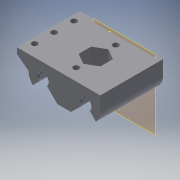
# Autodesk Inventor part: X Carriage
Saved by Autodesk Inventor 2016 (Build 200138000, 138)
## iProperties
Created: 2016-05-27
Part Number: X Carriage
Material: Generic
Document SubType Name: Modeling
Designer: Scott
Density: 1 g/cm^3
Appearance: Default
Author: Scott
Autodesk Inventor part; units mm, degrees
ref_plane "YZ Plane" through (0, 0, 0) normal (1, 0, 0) x (0, 1, 0)
ref_plane "XZ Plane" through (0, 0, 0) normal (0, 1, 0) x (-1, 0, 0)
ref_plane "XY Plane" through (0, 0, 0) normal (0, 0, 1) x (1, 0, 0)
ref_plane "Work Plane1" through (0, 0, 0) normal (0, 0, 1) x (1, 0, 0)
sketch "Sketch1" plane through (0, 0, 0) normal (0, 0, 1) x (1, 0, 0)
  circle A0 centre (31.455, -10.16) radius 4 projected
  circle A1 centre (-6.055, -10.16) radius 4 projected
  circle A2 centre (-6.055, -10.16) radius 8
  circle A3 centre (31.455, -10.16) radius 8
  circle A4 centre (-6.055, -10.16) radius 12.7
  circle A5 centre (31.455, -10.16) radius 12.7
  line L0 (-6.055, 2.54) -> (31.455, 2.54)
  line L1 (-6.055, -22.86) -> (31.455, -22.86)
  point P0 (0, 0)
  dimension "d0" = 16
  dimension "d1" = 16
  dimension "d2" = 25.4
  dimension "d3" = 25.4
  constraints: 4 centre point, 4 coincident, 4 end point, 4 point on circle, 2 tangent
  measures "d0" diameter of A2
  measures "d1" diameter of A3
  measures "d2" diameter of A4
  measures "d3" diameter of A5
extrude "Extrusion1" add sketch "Sketch1" along normal blind 24 contours A4 | A4 L0 A5 L1 | A5
sketch "Sketch2" plane through (-6.055, 2.54, 0) normal (0, 1, 0) x (1, 0, 0)
  point P0 (6.055, 0)
sketch "Sketch3" plane through (0, 0, 24) normal (0, 0, 1) x (1, 0, 0)
  circle A0 centre (31.455, -10.16) radius 8 projected
  circle A1 centre (-6.055, -10.16) radius 8 projected
  line L0 (-6.055, -22.86) -> (31.455, -22.86) projected
  arc A2 (31.455, -22.86) -> (31.455, 2.54) centre (31.455, -10.16) ccw projected
  line L1 (31.455, 2.54) -> (-6.055, 2.54) projected
  arc A3 (-6.055, 2.54) -> (-6.055, -22.86) centre (-6.055, -10.16) ccw projected
  circle A4 centre (-6.055, -10.16) radius 5
  circle A5 centre (31.455, -10.16) radius 5
  point P0 (0, 0)
  dimension "d6" = 10
  dimension "d7" = 10
  constraints: 2 centre point, 2 coincident
  measures "d6" diameter of A4
  measures "d7" diameter of A5
extrude "Extrusion2" add sketch "Sketch3" along normal blind 2 contours A0 | A1 | A3 L1 A2 L0
sketch "Sketch4" plane through (0, 0, 26) normal (0, 0, 1) x (1, 0, 0)
  circle A0 centre (-6.055, -10.16) radius 5 projected
  circle A1 centre (31.455, -10.16) radius 5 projected
  line L0 (-6.055, -22.86) -> (31.455, -22.86) projected
  arc A2 (31.455, -22.86) -> (31.455, 2.54) centre (31.455, -10.16) ccw projected
  line L1 (31.455, 2.54) -> (-6.055, 2.54) projected
  arc A3 (-6.055, 2.54) -> (-6.055, -22.86) centre (-6.055, -10.16) ccw projected
  circle A4 centre (-6.055, -10.16) radius 8 projected
  circle A5 centre (31.455, -10.16) radius 8 projected
  point P0 (0, 0)
extrude "Extrusion3" add sketch "Sketch4" along normal blind 24 contours A3 L1 A2 L0
sketch "Sketch5" plane through (-6.055, 2.54, 0) normal (0, 1, 0) x (1, 0, 0)
  line L0 (37.51, 0) -> (0, 0) projected
  line L1 (0, 0) -> (0, -50) projected
  line L2 (37.51, -50) -> (0, -50) projected
  line L3 (37.51, 0) -> (37.51, -50) projected
  circle A0 centre (18.755, -25) radius 6.5
  point P0 (6.055, 0)
  dimension "d12" = 13
  constraints: 1 centre point
  measures "d12" diameter of A0
extrude "Extrusion4" cut sketch "Sketch5" against normal blind 36.700003 contours A0
sketch "Sketch6" plane through (0, 0, 50) normal (0, 0, 1) x (1, 0, 0)
  circle A0 centre (31.455, -10.16) radius 8
  circle A1 centre (-6.055, -10.16) radius 8
  line L0 (-6.055, -22.86) -> (31.455, -22.86)
  arc A2 (31.455, -22.86) -> (31.455, 2.54) centre (31.455, -10.16) ccw
  line L1 (31.455, 2.54) -> (-6.055, 2.54)
  arc A3 (-6.055, 2.54) -> (-6.055, -22.86) centre (-6.055, -10.16) ccw
  circle A4 centre (-6.055, -10.16) radius 8
  line L2 (-11.774138, -15.753877) -> (-14.91362, -19.260266)
  arc A5 (-6.055, 2.54) -> (-6.055, -22.86) centre (-6.055, -10.16) ccw
  line L3 (-11.774138, -15.753877) -> (-7.067641, -15.753877) construction
  line L4 (-0.461123, -15.879138) -> (6.51974, -22.86)
  line L5 (-6.055, -22.86) -> (31.455, -22.86)
  line L6 (-0.461123, -15.879138) -> (9.411307, -15.879138) construction
  circle A6 centre (31.455, -10.16) radius 8
  line L7 (25.735862, -15.753877) -> (18.470616, -22.86)
  line L8 (37.048877, -15.879138) -> (40.33528, -19.239131)
  arc A7 (31.455, -22.86) -> (31.455, 2.54) centre (31.455, -10.16) ccw
  line L9 (25.735862, -15.753877) -> (31.455, -10.16)
  line L10 (31.455, -10.16) -> (37.048877, -15.879138)
  line L11 (-0.461123, -15.879138) -> (-6.055, -10.16)
  line L12 (-6.055, -10.16) -> (-11.774138, -15.753877)
  point P0 (0, 0)
  dimension "d16" = 45
  constraints: 20 end point, 11 point on circle, 4 perpendicular, 2 equal length, 2 horizontal, 2 point on line, 1 parallel
  measures "d16" angle of L4 L6
extrude "Extrusion5" cut sketch "Sketch6" against normal blind 96.8375 contours L9 L10 A0 | A0 L8 A2 L0 L7 | L0 A3 L2 A1 L4 | A1 L12 L11 picked at (31.396323, -15.459474) picked at (-8.407222, -14.909202)
sketch "Sketch7" plane through (0, 0, 0) normal (0, 0, -1) x (-1, 0, 0)
  line L0 (11.774138, -15.753877) -> (14.91362, -19.260266)
  arc A0 (14.91362, -19.260266) -> (6.055, 2.54) centre (6.055, -10.16) ccw
  line L1 (-31.455, 2.54) -> (6.055, 2.54)
  arc A1 (-31.455, 2.54) -> (-40.33528, -19.239131) centre (-31.455, -10.16) ccw
  line L2 (-40.33528, -19.239131) -> (-37.048877, -15.879138)
  arc A2 (-25.735862, -15.753877) -> (-37.048877, -15.879138) centre (-31.455, -10.16) ccw
  line L3 (-25.735862, -15.753877) -> (-18.470616, -22.86)
  line L4 (-6.51974, -22.86) -> (-18.470616, -22.86)
  line L5 (-6.51974, -22.86) -> (0.461123, -15.879138)
  arc A3 (11.774138, -15.753877) -> (0.461123, -15.879138) centre (6.055, -10.16) ccw
  arc A4 (-25.735862, -15.753877) -> (-37.048877, -15.879138) centre (-31.455, -10.16) ccw
  arc A5 (-27.880539, -13.656173) -> (-34.951173, -13.734461) centre (-31.455, -10.16) ccw
  line L6 (-37.048877, -15.879138) -> (-34.951173, -13.734461)
  arc A6 (-27.880539, -13.656173) -> (-34.951173, -13.734461) centre (-31.455, -10.16) ccw
  line L7 (-27.880539, -13.656173) -> (-25.735862, -15.753877)
  arc A7 (-25.735862, -15.753877) -> (-37.048877, -15.879138) centre (-31.455, -10.16) ccw
  line L8 (9.629461, -13.656173) -> (11.774138, -15.753877)
  arc A8 (11.774138, -15.753877) -> (0.461123, -15.879138) centre (6.055, -10.16) ccw
  line L9 (0.461123, -15.879138) -> (2.558827, -13.734461)
  arc A9 (9.629461, -13.656173) -> (2.558827, -13.734461) centre (6.055, -10.16) ccw
  point P0 (0, 0)
extrude "Extrusion6" add sketch "Sketch7" along normal blind 2.54
sketch "Sketch8" plane through (0, 0, 50) normal (0, 0, 1) x (1, 0, 0)
  line L0 (-14.91362, -19.260266) -> (-11.774138, -15.753877)
  arc A0 (-0.461123, -15.879138) -> (-11.774138, -15.753877) centre (-6.055, -10.16) ccw
  line L1 (-0.461123, -15.879138) -> (6.51974, -22.86)
  line L2 (6.51974, -22.86) -> (18.470616, -22.86)
  line L3 (18.470616, -22.86) -> (25.735862, -15.753877)
  arc A1 (37.048877, -15.879138) -> (25.735862, -15.753877) centre (31.455, -10.16) ccw
  line L4 (37.048877, -15.879138) -> (40.33528, -19.239131)
  arc A2 (40.33528, -19.239131) -> (31.455, 2.54) centre (31.455, -10.16) ccw
  line L5 (31.455, 2.54) -> (-6.055, 2.54)
  arc A3 (-6.055, 2.54) -> (-14.91362, -19.260266) centre (-6.055, -10.16) ccw
  line L6 (-11.774138, -15.753877) -> (-9.629461, -13.656173)
  arc A4 (-2.558827, -13.734461) -> (-9.629461, -13.656173) centre (-6.055, -10.16) ccw
  line L7 (-2.558827, -13.734461) -> (-0.461123, -15.879138)
  arc A5 (-0.461123, -15.879138) -> (-11.774138, -15.753877) centre (-6.055, -10.16) ccw
  line L8 (34.951173, -13.734461) -> (37.048877, -15.879138)
  arc A6 (37.048877, -15.879138) -> (25.735862, -15.753877) centre (31.455, -10.16) ccw
  line L9 (25.735862, -15.753877) -> (27.880539, -13.656173)
  arc A7 (34.951173, -13.734461) -> (27.880539, -13.656173) centre (31.455, -10.16) ccw
  point P0 (0, 0)
extrude "Extrusion7" add sketch "Sketch8" along normal blind 2.54
sketch "Sketch9" plane through (-6.055, 2.54, -2.54) normal (0, 1, 0) x (1, 0, 0)
  line L0 (50.21, 0) -> (50.21, -55.08) projected
  line L1 (37.51, 0) -> (37.51, -55.08) projected
  line L2 (50.21, 0) -> (37.51, 0) projected
  line L3 (37.51, -55.08) -> (50.21, -55.08) projected
  point P0 (6.055, -2.54)
  point P1 (46.39028, 0)
  point P2 (46.39028, -55.08)
extrude "Extrusion8" add sketch "Sketch9" against normal up to next
sketch "Sketch10" plane through (-6.055, 2.54, 52.54) normal (0, 1, 0) x (1, 0, 0)
  line L0 (5, 0) -> (-5, 0)
  line L1 (-8, 52.54) -> (8, 52.54)
  line L2 (-5.719138, 52.54) -> (-5.719138, 2.54)
  line L3 (-5.719138, 52.54) -> (44.280862, 52.54) construction
  circle A0 centre (18.755, 27.54) radius 6.5
  line L4 (0, 55.08) -> (0, 0)
  line L5 (50.21, 0) -> (0, 0)
  line L6 (50.21, 55.08) -> (50.21, 0)
  line L7 (0, 55.08) -> (50.21, 55.08)
  line L8 (-8.85862, 55.08) -> (-8.85862, 0)
  line L9 (0, 0) -> (-8.85862, 0)
  line L10 (0, 55.08) -> (0, 0)
  line L11 (-8.85862, 55.08) -> (0, 55.08)
  point P0 (6.055, 52.54)
  point P1 (-3.574461, 0)
  point P2 (3.496173, 0)
  point P3 (5.593877, 52.54)
  dimension "d25" = 90
  constraints: 4 end point, 1 horizontal, 1 perpendicular
  measures "d25" angle of L2 L3
extrude "Extrusion9" add sketch "Sketch10" against normal up to next contours L0 L9 L8 L11 L4
sketch "Sketch11" plane through (44.155, 2.54, 52.54) normal (0, 1, 0) x (1, 0, 0)
  line L0 (0, 55.08) -> (0, 0)
  line L1 (-4.7, 52.54) -> (-4.7, 28.54)
  line L2 (0, 55.08) -> (0, 0)
  line L3 (0, 0) -> (-59.06862, 0)
  line L4 (0, 55.08) -> (-3.81, 55.08)
  line L5 (-3.81, 55.08) -> (-3.81, 0)
  line L6 (-3.81, 0) -> (0, 0)
  line L7 (0, 0) -> (0, 55.08)
  point P0 (-44.155, 52.54)
  dimension "d28" = 3.81
  constraints: 8 end point, 2 parallel, 1 horizontal, 1 perpendicular, 1 point on line
  measures "d28" distance of L6.end L5.end
extrude "Extrusion10" add sketch "Sketch11" along normal blind 12.7
sketch "Sketch12" plane through (-14.91362, 2.54, 52.54) normal (0, 1, 0) x (1, 0, 0)
  line L0 (55.25862, 0) -> (55.25862, 55.08)
  line L1 (55.25862, 55.08) -> (0, 55.08)
  line L2 (0, 55.08) -> (0, 0)
  line L3 (55.25862, 0) -> (0, 0)
  circle A0 centre (27.61362, 27.54) radius 6.5
  circle A1 centre (27.61362, 27.54) radius 6.5
  line L4 (27.475496, 34.038532) -> (27.475496, 55.08)
  line L5 (33.384236, 55.08) -> (21.43336, 55.08)
  line L6 (27.475496, 34.038532) -> (48.516964, 34.038532) construction
  line L7 (27.478162, 21.041412) -> (27.478162, 0)
  line L8 (55.25862, 0) -> (0, 0)
  line L9 (27.478162, 21.041412) -> (48.519574, 21.041412) construction
  circle A2 centre (27.62931, 44.942828) radius 2.54
  circle A3 centre (27.478162, 10.520706) radius 2.54
  point P0 (14.91362, 52.54)
  dimension "d31" = 90
  dimension "d32" = 90
  dimension "d33" = 5.08
  dimension "d34" = 5.08
  constraints: 8 end point, 4 point on circle, 2 centre point, 2 horizontal, 2 perpendicular, 2 point on line, 1 midpoint
  measures "d31" angle of L6 L4
  measures "d32" angle of L7 L9
  measures "d33" diameter of A2
  measures "d34" diameter of A3
extrude "Extrusion11" cut sketch "Sketch12" against normal blind 76.2 contours A3 L7 | L7 A3 | A2 L4 | L4 A2
sketch "Sketch13" plane through (-14.91362, 2.54, 52.54) normal (0, 1, 0) x (1, 0, 0)
  line L0 (0, 0) -> (0, 55.08)
  line L1 (0, 55.08) -> (0, 55.08)
  line L2 (0, 55.08) -> (0, 0)
  line L3 (0, 0) -> (0, 0)
  line L4 (-3.84138, 55.08) -> (-3.84138, 0)
  line L5 (0, 55.08) -> (-3.84138, 55.08)
  line L6 (-3.84138, 55.08) -> (-3.84138, 0)
  line L7 (-3.84138, 0) -> (0, 0)
  line L8 (0, 0) -> (0, 55.08)
  point P0 (14.91362, 52.54)
  constraints: 8 end point, 2 parallel, 1 horizontal, 1 perpendicular
extrude "Extrusion12" add sketch "Sketch13" against normal up to surface
sketch "Sketch14" plane through (40.345, 2.54, 52.54) normal (0, 1, 0) x (1, 0, 0)
  circle A0 centre (-27.780458, 10.520706) radius 2.54
  circle A1 centre (-27.62931, 44.942828) radius 2.54
  line L0 (0, 0) -> (0, 55.08)
  line L1 (0, 55.08) -> (-59.1, 55.08)
  line L2 (-59.1, 55.08) -> (-59.1, 0)
  line L3 (0, 0) -> (-59.1, 0)
  circle A2 centre (-27.645, 27.54) radius 6.5
  line L4 (-59.1, 55.08) -> (-69.26, 55.08)
  line L5 (-69.26, 55.08) -> (-69.26, 0)
  line L6 (-69.26, 0) -> (-59.1, 0)
  line L7 (-59.1, 0) -> (-59.1, 55.08)
  point P0 (-40.345, 52.54)
  dimension "d39" = 10.16
  constraints: 8 end point, 2 parallel, 1 horizontal, 1 perpendicular
  measures "d39" distance of L6.end L5.end
extrude "Extrusion13" add sketch "Sketch14" against normal blind 5.08 contours L6 L5 L4 L2
sketch "Sketch15" plane through (0, 0, -2.54) normal (0, 0, -1) x (-1, 0, 0)
  line L0 (-40.345, 2.54) -> (28.915, 2.54)
  line L1 (-40.345, 2.54) -> (-40.345, 15.24)
  line L2 (-44.155, 15.24) -> (-40.345, 15.24)
  line L3 (-44.155, -10.16) -> (-44.155, 15.24)
  arc A0 (-44.155, -10.16) -> (-40.33528, -19.239131) centre (-31.455, -10.16) ccw
  line L4 (-40.33528, -19.239131) -> (-34.951173, -13.734461)
  arc A1 (-27.880539, -13.656173) -> (-34.951173, -13.734461) centre (-31.455, -10.16) ccw
  line L5 (-27.880539, -13.656173) -> (-18.470616, -22.86)
  line L6 (-18.470616, -22.86) -> (-6.51974, -22.86)
  line L7 (-6.51974, -22.86) -> (0.461123, -15.879138)
  line L8 (0.461123, -15.879138) -> (2.558827, -13.734461)
  arc A2 (9.629461, -13.656173) -> (2.558827, -13.734461) centre (6.055, -10.16) ccw
  line L9 (9.629461, -13.656173) -> (11.774138, -15.753877)
  line L10 (11.774138, -15.753877) -> (14.91362, -19.260266)
  arc A3 (14.91362, -19.260266) -> (18.755, -10.16) centre (6.055, -10.16) ccw
  line L11 (18.755, -2.54) -> (18.755, -10.16)
  line L12 (28.915, -2.54) -> (18.755, -2.54)
  line L13 (28.915, 2.54) -> (28.915, -2.54)
  line L14 (18.755, -2.54) -> (18.755, -10.16)
  line L15 (28.915, -2.54) -> (18.755, -2.54)
  line L16 (18.755, -10.16) -> (28.915, -2.54)
  point P0 (0, 0)
  constraints: 2 end point
extrude "Extrusion14" add sketch "Sketch15" against normal blind 2.54 contours L16 L11 L12
sketch "Sketch16" plane through (0, 0, 52.54) normal (0, 0, 1) x (1, 0, 0)
  line L0 (-18.755, -2.54) -> (-18.755, -10.16) projected
  line L1 (-18.755, -2.54) -> (-28.915, -2.54) projected
  line L2 (-18.755, -10.16) -> (-28.915, -2.54)
  point P0 (0, 0)
  constraints: 2 end point
extrude "Extrusion15" add sketch "Sketch16" against normal blind 2.54
sketch "Sketch17" plane through (40.345, 2.54, 52.54) normal (0, 1, 0) x (1, 0, 0)
  circle A0 centre (-27.780458, 10.520706) radius 2.54
  circle A1 centre (-27.62931, 44.942828) radius 2.54
  line L0 (0, 0) -> (0, 55.08)
  line L1 (0, 55.08) -> (-69.26, 55.08)
  line L2 (-69.26, 55.08) -> (-69.26, 0)
  line L3 (0, 0) -> (-69.26, 0)
  circle A2 centre (-27.645, 27.54) radius 6.5
  line L4 (-59.1, 2.54) -> (-59.1, 52.54)
  line L5 (-59.1, 55.08) -> (-59.1, 52.54)
  line L6 (-69.26, 52.54) -> (-59.1, 52.54)
  line L7 (-59.1, 52.54) -> (-69.26, 52.54)
  circle A3 centre (-64.18, 44.942828) radius 2.54
  circle A4 centre (-64.18, 10.520706) radius 2.54
  line L8 (-27.645, 27.54) -> (-64.18, 27.54)
  circle A5 centre (-64.18, 27.54) radius 2.54
  point P0 (-40.345, 52.54)
  dimension "d46" = 5.08
  dimension "d47" = 5.08
  dimension "d48" = 5.08
  constraints: 4 end point, 3 centre point, 1 coincident, 1 collinear, 1 horizontal
  measures "d46" diameter of A3
  measures "d47" diameter of A4
  measures "d48" diameter of A5
extrude "Extrusion16" cut sketch "Sketch17" against normal blind 13.6525 contours A3 | A4 | A5
sketch "Sketch18" plane through (40.345, 2.54, 52.54) normal (0, 1, 0) x (1, 0, 0)
  circle A0 centre (-64.18, 10.520706) radius 2.54
  circle A1 centre (-64.18, 44.942828) radius 2.54
  circle A2 centre (-64.18, 27.54) radius 2.54
  circle A3 centre (-27.780458, 10.520706) radius 2.54
  circle A4 centre (-27.62931, 44.942828) radius 2.54
  line L0 (0, 0) -> (0, 55.08)
  line L1 (0, 55.08) -> (-69.26, 55.08)
  line L2 (-69.26, 55.08) -> (-69.26, 0)
  line L3 (0, 0) -> (-69.26, 0)
  circle A5 centre (-27.645, 27.54) radius 6.5
  line L4 (0, 0) -> (0, 55.08)
  line L5 (0, 55.08) -> (3.81, 55.08)
  line L6 (3.81, 55.08) -> (3.81, 0)
  line L7 (3.81, 0) -> (0, 0)
  line L8 (0, 0) -> (0, 55.08)
  point P0 (-40.345, 52.54)
  constraints: 8 end point, 2 parallel, 1 horizontal, 1 perpendicular
extrude "Extrusion17" cut sketch "Sketch18" along normal blind 25.4 contours L0 L5 L6 L7
sketch "Sketch19" plane through (44.155, 2.54, 52.54) normal (0, 1, 0) x (1, 0, 0)
  circle A0 centre (-67.99, 10.520706) radius 2.54
  circle A1 centre (-67.99, 44.942828) radius 2.54
  circle A2 centre (-67.99, 27.54) radius 2.54
  circle A3 centre (-31.590458, 10.520706) radius 2.54
  circle A4 centre (-31.43931, 44.942828) radius 2.54
  line L0 (0, 55.08) -> (-73.07, 55.08)
  line L1 (-73.07, 55.08) -> (-73.07, 0)
  line L2 (0, 0) -> (-73.07, 0)
  line L3 (0, 55.08) -> (0, 0)
  circle A5 centre (-31.455, 27.54) radius 6.5
  line L4 (-31.455, 38.509655) -> (-21.955, 33.024828)
  line L5 (-21.955, 33.024828) -> (-21.955, 22.055172)
  line L6 (-21.955, 22.055172) -> (-31.455, 16.570345)
  line L7 (-31.455, 16.570345) -> (-40.955, 22.055172)
  line L8 (-40.955, 22.055172) -> (-40.955, 33.024828)
  line L9 (-40.955, 33.024828) -> (-31.455, 38.509655)
  point P0 (-44.155, 52.54)
  dimension "d53" = 19
  constraints: 12 end point, 1 coincident, 13 other
  measures "d53" distance between parallel lines of L8 L5
extrude "Extrusion18" cut sketch "Sketch19" against normal blind 20.32 contours L4 L5 L6 L7 L8 L9
sketch "Sketch20" plane through (6.51974, -22.86, -2.54) normal (0, -1, 0) x (1, 0, 0)
  circle A0 centre (6.19595, 10.137172) radius 2.54
  circle A1 centre (6.044802, 44.559294) radius 2.54
  circle A2 centre (6.19595, 10.137172) radius 5.08
  circle A3 centre (6.044802, 44.559294) radius 5.08
  point P0 (-6.51974, 2.54)
  dimension "d56" = 10.16
  dimension "d57" = 10.16
  constraints: 2 centre point, 2 coincident
  measures "d56" diameter of A2
  measures "d57" diameter of A3
extrude "Extrusion19" cut sketch "Sketch20" against normal blind 12.7
fillet "Fillet1" radius 4.7625 4 edges at (25.7359, -15.7539, 12) (25.7359, -15.7539, 38) (37.0489, -15.8791, 38) (37.0489, -15.8791, 12)
fillet "Fillet2" radius 4.7625 4 edges at (-11.7741, -15.7539, 12) (-0.4611, -15.8791, 12) (-0.4611, -15.8791, 38) (-11.7741, -15.7539, 38)
sketch "Sketch21" plane through (0, 0, 50) normal (0, 0, -1) x (-1, 0, 0)
  arc A0 (13.382373, -13.370858) -> (-1.280528, -13.352182) centre (6.055, -10.16) ccw
  arc A1 (-2.279864, -18.620124) -> (-1.280528, -13.352182) centre (-5.64746, -15.252528) ccw
  line L0 (-2.279864, -18.620124) -> (0.461123, -15.879138)
  line L1 (2.558827, -13.734461) -> (0.461123, -15.879138)
  arc A2 (9.629461, -13.656173) -> (2.558827, -13.734461) centre (6.055, -10.16) ccw
  line L2 (9.629461, -13.656173) -> (13.499513, -17.441463)
  arc A3 (13.382373, -13.370858) -> (13.499513, -17.441463) centre (17.744449, -15.282322) ccw
  arc A4 (-24.06155, -13.215633) -> (-38.778981, -13.378588) centre (-31.455, -10.16) ccw
  arc A5 (-39.734364, -18.624759) -> (-38.778981, -13.378588) centre (-43.139038, -15.294654) ccw
  line L3 (-39.734364, -18.624759) -> (-34.951173, -13.734461)
  arc A6 (-27.880539, -13.656173) -> (-34.951173, -13.734461) centre (-31.455, -10.16) ccw
  line L4 (-27.880539, -13.656173) -> (-22.990241, -18.439364)
  arc A7 (-24.06155, -13.215633) -> (-22.990241, -18.439364) centre (-19.660136, -15.034689) ccw
  circle A8 centre (6.055, -10.16) radius 8.5
  circle A9 centre (-31.455, -10.16) radius 8.5
  point P0 (0, 0)
  dimension "d62" = 17
  dimension "d63" = 17
  constraints: 2 centre point, 2 coincident
  measures "d62" diameter of A8
  measures "d63" diameter of A9
extrude "Extrusion20" cut sketch "Sketch21" along normal up to surface (50 mm away) contours A3 A8 L2 A2 L1 L0 A1 A0 | A0 A1 A8 A3 | A8 L0 L1 A2 L2 | A7 A9 L4 A6 L3 A5 A4 | A4 A5 A9 A7 | A9 L3 A6 L4
body "Solid1"
